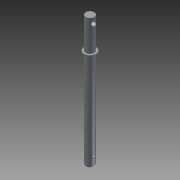
# Autodesk Inventor part: launcher.RBFpin
Saved by Autodesk Inventor 2011 (Build 150239000, 239)
## iProperties
Created: 2011-04-05
Part Number: launcher.RBFpin
Document SubType Name: Modeling
Designer: Rob
Density: 1 g/cm^3
Author: Rob
Autodesk Inventor part; units mm, degrees
ref_plane "XZ Plane" through (0, 0, 0) normal (0, 1, 0) x (-1, 0, 0)
ref_plane "XY Plane" through (0, 0, 0) normal (0, 0, 1) x (1, 0, 0)
sketch "Sketch1" plane through (0, 0, 0) normal (0, 0, 1) x (1, 0, 0)
  circle A0 centre (0, 0) radius 2.38125
  dimension "d0" = 4.7625
  constraints: 1 centre point, 1 coincident
  measures "d0" diameter of A0
extrude "Extrusion1" add sketch "Sketch1" along normal blind 73.3298
ref_plane "Work Plane1" through (5, 0, 0) normal (1, 0, 0) x (0, 1, 0)
sketch "Sketch2" plane through (5, 0, 0) normal (1, 0, 0) x (0, 1, 0)
  line L0 (-2.38125, 73.3298) -> (2.38125, 73.3298)
  line L1 (-2.38125, 0) -> (2.38125, 0)
  line L2 (-2.38125, 0) -> (-2.38125, 73.3298)
  line L3 (2.38125, 0) -> (2.38125, 73.3298)
  circle A0 centre (0, 70.142643) radius 1.35
  point P0 (0, 0)
  dimension "d4" = 2.7
  constraints: 1 centre point
  measures "d4" diameter of A0
extrude "Extrusion2" cut sketch "Sketch2" against normal blind 39.4202 contours A0
sketch "Sketch3" plane through (0, 0, 0) normal (1, 0, 0) x (0, 1, 0)
  arc A0 (-1.35, 70.142643) -> (-1.35, 70.142643) centre (-1.35, 70.142643) ccw
  arc A1 (-1.35, 70.142643) -> (-1.35, 70.142643) centre (-1.35, 70.142643) ccw
  line L0 (-2.38125, 73.3298) -> (2.38125, 73.3298)
  line L1 (-2.38125, 0) -> (2.38125, 0)
  line L2 (2.38125, 0) -> (2.38125, 73.3298)
  line L3 (-2.38125, 0) -> (-2.38125, 73.3298)
  line L4 (2.38125, 55.88) -> (3.38125, 55.88)
  line L5 (3.38125, 55.88) -> (3.38125, 55.38)
  line L6 (3.38125, 55.38) -> (2.38125, 55.38)
  line L7 (2.38125, 55.38) -> (2.38125, 55.88)
  line L8 (0, -14.66596) -> (0, 87.99576)
  point P0 (0, 0)
  dimension "d7" = 1
  dimension "d8" = 0.5
  dimension "d9" = 17.4498
  constraints: 8 end point, 2 parallel, 1 horizontal, 1 perpendicular, 1 point on line, 2 other
  measures "d7" distance of L5.end L6.end
  measures "d8" distance of L4.end L5.end
  measures "d9" distance between parallel lines of L0 L4
sketch "Sketch3 outline for Revolution1" plane through (0, 0, 0) normal (1, 0, 0) x (0, 1, 0)
  line L0 (3.38125, 55.88) -> (2.38125, 55.88)
  line L1 (3.38125, 55.38) -> (3.38125, 55.88)
  line L2 (2.38125, 55.38) -> (3.38125, 55.38)
  line L3 (2.38125, 55.88) -> (2.38125, 55.38)
revolve "Revolution1" add sketch "Sketch3 outline for Revolution1" angle 360 about axis through (0, 0, -10) along (0, 0, 1)
sketch "Sketch4" plane through (0, 0, 0) normal (1, 0, 0) x (0, 1, 0)
  circle A0 centre (0, 5.08) radius 0.7
  point P0 (0, 0)
  dimension "d11" = 1.4
  dimension "d12" = 5.08
  constraints: 1 centre point
  measures "d11" diameter of A0
  measures "d12" distance of point (0, 0) A0.centre
extrude "Extrusion3" add sketch "Sketch4" along normal blind 2.9202
fillet "Fillet1" radius 0.6 1 edges at (2.9202, -0.7, 5.08)
fillet "Fillet2" radius 1.5 1 edges at (-2.3813, 0, 0)
body "Solid1"
